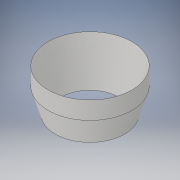
# Autodesk Inventor part: conic_reflector_5
Saved by Autodesk Inventor 2017 (Build 210142000, 142)
## iProperties
Created: 2017-07-10
Part Number: conic_reflector_5
Material: Generic
Document SubType Name: Modeling
Designer: richp
Density: 1 g/cm^3
Appearance: Default
Author: richp
Autodesk Inventor part; units mm, degrees
ref_plane "YZ Plane" through (0, 0, 0) normal (1, 0, 0) x (0, 1, 0)
ref_plane "XZ Plane" through (0, 0, 0) normal (0, 1, 0) x (-1, 0, 0)
ref_plane "XY Plane" through (0, 0, 0) normal (0, 0, 1) x (1, 0, 0)
sketch "Sketch1" plane through (0, 0, 0) normal (0, 0, 1) x (1, 0, 0)
  line L0 (0, -0.52) -> (0, 3.12) projected
  line L1 (-2.15, 0) -> (-2.6, 1.5)
  line L2 (-2.6, 1.5) -> (-2.6, 2.6)
  line L3 (-2.6, 2.6) -> (-1.82, 0)
  line L4 (-2.15, 0) -> (-1.82, 0)
  point P0 (0, 0)
  dimension "d15" = 2.6
  dimension "d16" = 2.15
  dimension "d17" = 2.6
  dimension "d18" = 1.1
  dimension "d19" = 16.699
  constraints: 8 end point, 1 horizontal, 1 horizontal alignment, 1 parallel, 1 vertical
  measures "d15" horizontal distance of point (0, 0) L2.end
  measures "d16" distance of point (0, 0) L1.start
  measures "d17" distance between parallel lines of L0 L2
  measures "d18" distance of L1.end L2.end
  measures "d19" angle of L0 L3
revolve "Revolution1" add sketch "Sketch1" angle 360 about axis through (0, -10, 0) along (0, 1, 0)
body "Solid1"
